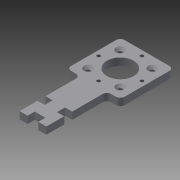
# Autodesk Inventor part: pitch_mount
Saved by Autodesk Inventor 2015 (Build 190159000, 159)
## iProperties
Created: 2015-12-01
Part Number: pitch_mount
Material: Generic
Document SubType Name: Modeling
Designer: jufranz
Density: 1 g/cm^3
Appearance: Default
Author: jufranz
Autodesk Inventor part; units mm, degrees
ref_plane "YZ Plane" through (0, 0, 0) normal (1, 0, 0) x (0, 1, 0)
ref_plane "XZ Plane" through (0, 0, 0) normal (0, 1, 0) x (-1, 0, 0)
ref_plane "XY Plane" through (0, 0, 0) normal (0, 0, 1) x (1, 0, 0)
sketch "Sketch1" plane through (0, 0, 0) normal (0, 1, 0) x (-1, 0, 0)
  line L0 (20, 16.825) -> (20, -16.825)
  line L1 (16.825, -20) -> (-16.825, -20)
  line L2 (-20, -16.825) -> (-20, 16.825)
  line L3 (-16.825, 20) -> (-13.175, 20)
  line L4 (-10, 23.175) -> (-10, 60)
  line L5 (-10, 60) -> (10, 60)
  line L6 (10, 60) -> (10, 23.175)
  line L7 (13.175, 20) -> (16.825, 20)
  arc A0 (10, 23.175) -> (13.175, 20) centre (13.175, 23.175) ccw
  arc A1 (-13.175, 20) -> (-10, 23.175) centre (-13.175, 23.175) ccw
  arc A2 (20, 16.825) -> (16.825, 20) centre (16.825, 16.825) ccw
  arc A3 (16.825, -20) -> (20, -16.825) centre (16.825, -16.825) ccw
  arc A4 (-20, -16.825) -> (-16.825, -20) centre (-16.825, -16.825) ccw
  arc A5 (-16.825, 20) -> (-20, 16.825) centre (-16.825, 16.825) ccw
  point P0 (0, 0)
  point P1 (20, 20)
  point P2 (20, -20)
  point P3 (-20, -20)
  point P4 (-20, 20)
  point P5 (-10, 20)
  point P6 (10, 20)
  point P7 (20, 0)
  point P8 (0, -20)
  point P9 (0, 60)
  dimension "d0" = 40
  dimension "d1" = 40
  dimension "d2" = 20
  dimension "d3" = 60
  dimension "d26" = 3.175
  dimension "d27" = 3.175
  constraints: 16 end point, 13 point on line, 12 point on circle, 12 tangent, 7 perpendicular, 6 centre point, 4 equal radius, 3 midpoint, 2 vertical alignment, 1 horizontal alignment, 1 vertical
  measures "d0" distance of point (20, 20) point (20, -20)
  measures "d1" distance of point (20, -20) point (-20, -20)
  measures "d2" distance between parallel lines of L4 L6
  measures "d3" distance from line of point (0, 0) L5
  measures "d26" radius of A0
  measures "d27" radius of A2
extrude "Extrusion1" add sketch "Sketch1" along normal blind 5.334
sketch "Sketch2" plane through (0, 5.334, 0) normal (0, 1, 0) x (1, 0, 0)
  line L0 (-12.0208, -12.0208) -> (0, 0)
  line L1 (0, 0) -> (-20, 0)
  line L2 (-20, 16.825) -> (-20, -16.825) projected
  point P0 (-17.5, 17.5)
  point P1 (-17.5, -17.5)
  point P2 (12.0208, -12.0208)
  point P3 (12.0208, 12.0208)
  point P4 (-12.0208, 12.0208)
  dimension "d6" = 17
  dimension "d7" = 45
  dimension "d10" = 360
  constraints: 4 end point, 1 coincident, 7 other
  measures "d6" distance of point (0, 0) L0.start
  measures "d7" angle of L0 L1
hole "Hole1" at (-12.0208, 5.334, 12.0208) at (12.0208, 5.334, 12.0208) at (12.0208, 5.334, -12.0208) at (-12.0208, 5.334, -12.0208) direction (0, -1, 0) diameter 3.2 end through all countersink diameter 6.35 countersink angle 82
sketch "Sketch3" plane through (0, 5.334, 0) normal (0, 1, 0) x (1, 0, 0)
  point P0 (0, 0)
  point P1 (0, 0)
  constraints: 1 coincident
hole "Hole2" at (0, 5.334, 0) direction (0, -1, 0) diameter 20 end through all
sketch "Sketch4" plane through (0, 5.334, 0) normal (0, 1, 0) x (1, 0, 0)
  point P0 (0, 0)
  point P1 (-16.215, 0)
  point P2 (0, -16.215)
  point P3 (16.215, 0)
  point P4 (0, 16.215)
  dimension "d29" = 16.215
  dimension "d47" = 360
  constraints: 5 other
  measures "d29" distance of point (-16.215, 0) point (0, 0)
hole "Hole3" at (-16.215, 5.334, 0) at (0, 5.334, 16.215) at (16.215, 5.334, 0) at (0, 5.334, -16.215) direction (0, -1, 0) diameter 2.4638 end through all
sketch "Sketch6" plane through (10, 0, 60) normal (1, 0, 0) x (0, 0, -1)
  line L0 (0, 5.334) -> (36.825, 5.334) projected
  line L1 (0, 0) -> (36.825, 0) projected
  line L2 (14, 5.334) -> (8, 5.334)
  line L3 (8, 5.334) -> (8, 0)
  line L4 (8, 0) -> (14, 0)
  line L5 (14, 0) -> (14, 5.334)
  line L6 (0, 0) -> (0, 5.334) projected
  point P0 (60, 0)
  dimension "d41" = 6
  dimension "d42" = 8
  constraints: 8 end point, 2 parallel, 2 point on line, 1 horizontal, 1 perpendicular
  measures "d41" distance between parallel lines of L3 L5
  measures "d42" distance between parallel lines of L6 L3
extrude "Extrusion3" cut sketch "Sketch6" against normal blind 5.334 contours L0 L5 L1 L3
sketch "Sketch5" plane through (-10, 0, 60) normal (0, 0, 1) x (1, 0, 0)
  line L0 (26.825, 0) -> (-6.825, 0) projected
  line L1 (20, 5.334) -> (14, 5.334)
  line L2 (14, 5.334) -> (14, 0)
  line L3 (14, 0) -> (20, 0)
  line L4 (20, 0) -> (20, 5.334)
  line L5 (0, 5.334) -> (20, 5.334) projected
  line L6 (0, 0) -> (6, 0)
  line L7 (6, 0) -> (6, 5.334)
  line L8 (6, 5.334) -> (0, 5.334)
  line L9 (0, 5.334) -> (0, 0)
  point P0 (10, 0)
  dimension "d37" = 6
  dimension "d38" = 6
  constraints: 16 end point, 4 parallel, 2 horizontal, 2 perpendicular, 2 point on line
  measures "d37" distance between parallel lines of L9 L7
  measures "d38" distance between parallel lines of L4 L2
extrude "Extrusion2" add sketch "Sketch5" along normal blind 5.334 contours L0 L2 L1 L4 | L0 L9 L5 L7
mirror "Mirror1" about plane through (0, 0, 0) normal (1, 0, 0) of "Extrusion3"
equation "\"d38\" = d37"
body "Solid1"
